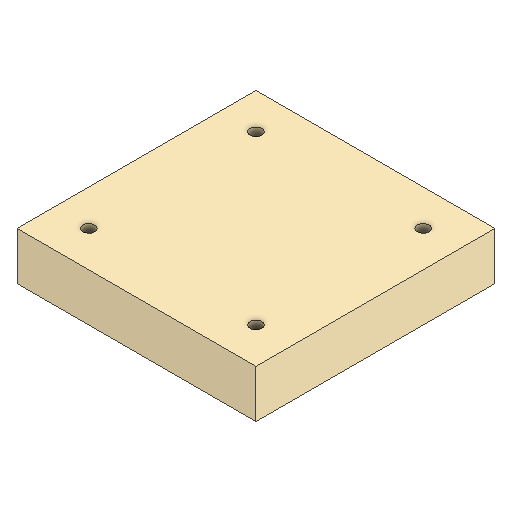
# Autodesk Inventor part: Plataforma
Saved by Autodesk Inventor 2026.1 (Build 301233000, 233)
## iProperties
Created: 2025-04-13
Part Number: Plataforma
Material: Genérico
Document SubType Name: Modeling
Designer: piero
Density: 1 g/cm^3
Appearance: Valor por defecto
Author: piero
Autodesk Inventor part; units mm, degrees
ref_plane "YZ Plane" through (0, 0, 0) normal (1, 0, 0) x (0, 1, 0)
ref_plane "XZ Plane" through (0, 0, 0) normal (0, 1, 0) x (-1, 0, 0)
ref_plane "Plano de trabajo2" through (0, 0, -500) normal (0, 0, 1) x (1, 0, 0)
sketch "Boceto2" plane through (0, 0, -500) normal (0, 0, 1) x (1, 0, 0)
  line L0 (400, 250) -> (500, 250)
  line L1 (500, 250) -> (500, 270)
  line L2 (500, 270) -> (400, 270)
  line L3 (400, 270) -> (400, 250)
  line L4 (150, 50) -> (150, 550) projected
  line L5 (0, 50) -> (1000, 50) projected
  line L6 (850, 50) -> (850, 550) projected
  point P0 (0, 0)
  dimension "d4" = 100
  dimension "d5" = 20
  dimension "d6" = 250
  dimension "d7" = 200
  dimension "d8" = 350
  constraints: 8 end point, 2 parallel, 1 horizontal, 1 perpendicular
  measures "d4" distance of L2.end L1.end
  measures "d5" distance of L1.end L0.end
  measures "d6" distance between parallel lines of L4 L3
  measures "d7" distance between parallel lines of L5 L0
  measures "d8" distance between parallel lines of L6 L1
extrude "Extrusión1" add sketch "Boceto2" along normal blind 50 and the other way blind 50
sketch "Boceto3" plane through (400, 270, -450) normal (0, 1, 0) x (1, 0, 0)
  circle A0 centre (15, 15) radius 2.5
  circle A1 centre (15, 85) radius 2.5
  circle A2 centre (85, 85) radius 2.5
  circle A3 centre (85, 15) radius 2.5
  line L0 (0, 100) -> (0, 0) projected
  line L1 (100, 100) -> (100, 0) projected
  line L2 (0, 100) -> (100, 100) projected
  line L3 (100, 0) -> (0, 0) projected
  point P0 (-400, -450)
  dimension "d13" = 5
  dimension "d14" = 5
  dimension "d15" = 5
  dimension "d16" = 5
  dimension "d17" = 15
  dimension "d18" = 15
  dimension "d19" = 15
  dimension "d20" = 15
  dimension "d21" = 15
  dimension "d22" = 15
  dimension "d23" = 15
  dimension "d24" = 15
  constraints: 4 centre point
  measures "d13" diameter of A0
  measures "d14" diameter of A1
  measures "d15" diameter of A2
  measures "d16" diameter of A3
  measures "d17" distance from line of L0 A0.centre
  measures "d18" distance from line of L0 A1.centre
  measures "d19" distance from line of L1 A2.centre
  measures "d20" distance from line of L1 A3.centre
  measures "d21" distance from line of L2 A1.centre
  measures "d22" distance from line of A2.centre L2
  measures "d23" distance from line of L3 A0.centre
  measures "d24" distance from line of L3 A3.centre
hole "Agujero1" at (485, 270, -465) direction (0, -1, 0) diameter 5 depth 5 tip angle 118
hole "Agujero2" at (415, 270, -465) direction (0, -1, 0) diameter 5 depth 5 tip angle 118
hole "Agujero3" at (415, 270, -535) direction (0, -1, 0) diameter 5 depth 5 tip angle 118
hole "Agujero4" at (485, 270, -535) direction (0, -1, 0) diameter 5 depth 5 tip angle 118
